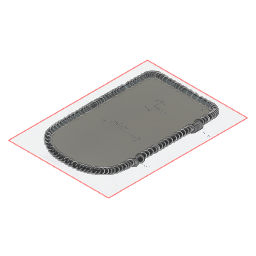
Uprint SE Screen (Autodesk Fusion 360 design; units mm, degrees)
Autodesk Fusion 360 part; units mm, degrees
sketch "Sketch1" plane through (0, 0, 0) normal (0, 0, 1) x (1, 0, 0)
  spline S0 degree 5 poles (-58.9, 25) (-58.8991, 25.1061) (-58.8974, 25.3171) (-58.8955, 25.6302) (-58.8941, 26.0406) (-58.8945, 26.5424) (-58.8966, 27.0343) (-58.9, 27.5189) (-58.9039, 28.0007) (-58.9072, 28.4862) (-58.9085, 28.9828) (-58.9065, 29.4974) (-58.9005, 30.0352) (-58.89, 30.598) (-58.8752, 31.1836) (-58.8572, 31.7866) (-58.8371, 32.4001) (-58.8162, 33.0168) (-58.7955, 33.6305) (-58.7759, 34.2371) (-58.7577, 34.8358) (-58.7409, 35.4283) (-58.725, 36.0179) (-58.7098, 36.6088) (-58.6948, 37.2055) (-58.6796, 37.8119) (-58.664, 38.431) (-58.648, 39.0645) (-58.6317, 39.7131) (-58.6152, 40.3763) (-58.5986, 41.052) (-58.5823, 41.7369) (-58.5663, 42.4263) (-58.5507, 43.1148) (-58.5357, 43.7974) (-58.5213, 44.4704) (-58.5075, 45.1325) (-58.4941, 45.7852) (-58.4811, 46.4341) (-58.468, 47.0889) (-58.4547, 47.7617) (-58.4408, 48.465) (-58.4259, 49.2109) (-58.41, 50.0087) (-58.3927, 50.8643) (-58.374, 51.7776) (-58.3541, 52.7428) (-58.3331, 53.7495) (-58.3114, 54.784) (-58.2892, 55.8308) (-58.2669, 56.8734) (-58.245, 57.8958) (-58.2238, 58.8838) (-58.2036, 59.8262) (-58.1848, 60.7157) (-58.1675, 61.5508) (-58.152, 62.335) (-58.1381, 63.0753) (-58.1258, 63.7812) (-58.1149, 64.4636) (-58.105, 65.134) (-58.0958, 65.8026) (-58.0865, 66.4778) (-58.0763, 67.1655) (-58.0646, 67.8691) (-58.0505, 68.59) (-58.0335, 69.3277) (-58.0133, 70.0802) (-57.9898, 70.8439) (-57.9634, 71.614) (-57.935, 72.385) (-57.9056, 73.1508) (-57.8763, 73.9064) (-57.848, 74.6475) (-57.8215, 75.3718) (-57.797, 76.0795) (-57.7742, 76.7738) (-57.7519, 77.4617) (-57.7287, 78.1521) (-57.7029, 78.8535) (-57.6729, 79.5733) (-57.6376, 80.3151) (-57.5967, 81.0775) (-57.5509, 81.8521) (-57.5019, 82.6224) (-57.4523, 83.3673) (-57.4046, 84.0651) (-57.3604, 84.697) (-57.3203, 85.2508) (-57.283, 85.7243) (-57.2445, 86.1299) (-57.1983, 86.4936) (-57.1374, 86.8447) (-57.0551, 87.2099) (-56.9468, 87.6027) (-56.8104, 88.0233) (-56.6459, 88.4642) (-56.4556, 88.9133) (-56.2433, 89.3591) (-56.0145, 89.7937) (-55.7743, 90.2123) (-55.5264, 90.6131) (-55.2717, 90.9968) (-55.0062, 91.367) (-54.7219, 91.729) (-54.4103, 92.0876) (-54.0646, 92.4458) (-53.6834, 92.803) (-53.273, 93.1523) (-52.8457, 93.4836) (-52.4159, 93.7859) (-51.9969, 94.0505) (-51.5979, 94.2734) (-51.2203, 94.4589) (-50.8589, 94.617) (-50.5057, 94.7597) (-50.1522, 94.897) (-49.7935, 95.0325) (-49.4276, 95.1645) (-49.0539, 95.2878) (-48.6727, 95.3967) (-48.283, 95.4865) (-47.8829, 95.5546) (-47.4692, 95.6002) (-47.0375, 95.6245) (-46.5821, 95.6312) (-46.0967, 95.6255) (-45.5763, 95.6131) (-45.018, 95.5995) (-44.4229, 95.5887) (-43.7967, 95.5829) (-43.1487, 95.5823) (-42.4895, 95.5859) (-41.8296, 95.592) (-41.1776, 95.5987) (-40.5384, 95.6041) (-39.9114, 95.6075) (-39.2909, 95.6084) (-38.6684, 95.6073) (-38.0341, 95.6047) (-37.3782, 95.6016) (-36.6931, 95.5986) (-35.975, 95.5963) (-35.2244, 95.5951) (-34.4448, 95.5949) (-33.6424, 95.5955) (-32.8245, 95.5967) (-31.9988, 95.5983) (-31.1729, 95.5998) (-30.3528, 95.601) (-29.5422, 95.6018) (-28.7429, 95.6021) (-27.955, 95.602) (-27.1781, 95.6016) (-26.4112, 95.601) (-25.6539, 95.6004) (-24.9064, 95.5999) (-24.1708, 95.5996) (-23.4507, 95.5995) (-22.7508, 95.5995) (-22.0753, 95.5997) (-21.4272, 95.5998) (-20.8072, 95.6) (-20.2126, 95.6) (-19.6359, 95.6) (-19.0653, 95.5999) (-18.4875, 95.5998) (-17.8893, 95.5998) (-17.2605, 95.5999) (-16.5953, 95.6001) (-15.8952, 95.6004) (-15.1686, 95.6008) (-14.4278, 95.601) (-13.6868, 95.601) (-12.9593, 95.6008) (-12.2558, 95.6003) (-11.582, 95.5996) (-10.9355, 95.5987) (-10.3068, 95.5979) (-9.6818, 95.5975) (-9.0444, 95.5977) (-8.3784, 95.5985) (-7.6701, 95.6002) (-6.911, 95.6026) (-6.0991, 95.6053) (-5.2378, 95.608) (-4.3344, 95.6102) (-3.3988, 95.6114) (-2.4427, 95.611) (-1.4776, 95.6086) (-0.5141, 95.6041) (0.4394, 95.5971) (1.3784, 95.5879) (2.3025, 95.5767) (3.2141, 95.5642) (4.1179, 95.5509) (5.0199, 95.5375) (5.9262, 95.5248) (6.8428, 95.5134) (7.7742, 95.5038) (8.7225, 95.4964) (9.687, 95.4914) (10.6632, 95.4887) (11.6446, 95.4879) (12.6231, 95.4888) (13.59, 95.4909) (14.537, 95.4935) (15.4567, 95.4963) (16.3436, 95.4987) (17.1952, 95.5005) (18.0128, 95.5015) (18.8017, 95.5018) (19.5702, 95.5014) (20.3282, 95.5008) (21.0862, 95.5001) (21.854, 95.4996) (22.6393, 95.4997) (23.4469, 95.5003) (24.2771, 95.5013) (25.1257, 95.5027) (25.9855, 95.5039) (26.8472, 95.5047) (27.7003, 95.5047) (28.5345, 95.5038) (29.3406, 95.5018) (30.1117, 95.4989) (30.8441, 95.4957) (31.538, 95.4929) (32.1959, 95.4912) (32.8216, 95.4916) (33.4196, 95.4943) (33.9936, 95.4995) (34.5453, 95.5063) (35.0741, 95.5132) (35.5782, 95.5177) (36.0567, 95.5163) (36.5115, 95.5039) (36.9493, 95.4745) (37.3833, 95.4202) (37.8291, 95.333) (38.3017, 95.2056) (38.8111, 95.0327) (39.3585, 94.8124) (39.935, 94.5462) (40.5255, 94.2385) (41.1116, 93.8957) (41.6747, 93.5252) (42.1988, 93.1351) (42.6737, 92.7332) (43.0977, 92.3261) (43.4746, 91.9191) (43.812, 91.5158) (44.1187, 91.1171) (44.4032, 90.7213) (44.6708, 90.3232) (44.9238, 89.9156) (45.1622, 89.4916) (45.385, 89.0467) (45.5901, 88.5811) (45.776, 88.102) (45.9413, 87.6203) (46.085, 87.1473) (46.2066, 86.6909) (46.3064, 86.2521) (46.3854, 85.8217) (46.4451, 85.385) (46.488, 84.9274) (46.5174, 84.4389) (46.5373, 83.9205) (46.5522, 83.3834) (46.5666, 82.8427) (46.5844, 82.3125) (46.6083, 81.8007) (46.6394, 81.303) (46.6765, 80.8014) (46.7175, 80.2727) (46.7595, 79.6944) (46.7993, 79.0515) (46.8342, 78.3428) (46.8624, 77.5884) (46.883, 76.8218) (46.896, 76.0823) (46.902, 75.407) (46.9025, 74.8232) (46.8993, 74.3408) (46.8949, 73.9426) (46.8923, 73.5835) (46.894, 73.209) (46.9016, 72.7699) (46.9155, 72.2407) (46.9341, 71.628) (46.955, 70.9576) (46.9753, 70.266) (46.9921, 69.5896) (47.0034, 68.956) (47.0086, 68.3729) (47.0085, 67.8217) (47.0053, 67.2706) (47.0015, 66.6843) (46.9991, 66.0356) (46.9997, 65.3148) (47.0031, 64.5426) (47.0074, 63.7742) (47.0102, 63.0768) (47.0093, 62.5129) (47.0042, 62.1193) (46.9969, 61.8927) (46.9928, 61.7611) (47.0033, 61.6066) (47.0613, 61.4198) (47.1962, 61.277) (47.3618, 61.2248) (47.5085, 61.2586) (47.6834, 61.3051) (47.9192, 61.3124) (48.1786, 61.2985) (48.4167, 61.2947) (48.6267, 61.3024) (48.8271, 61.3015) (49.0325, 61.2679) (49.2464, 61.1849) (49.4586, 61.0601) (49.6507, 60.9219) (49.8171, 60.7893) (49.9778, 60.6523) (50.1486, 60.4921) (50.3103, 60.302) (50.4273, 60.0853) (50.4851, 59.8481) (50.499, 59.5958) (50.4927, 59.3302) (50.4827, 59.0468) (50.4778, 58.7398) (50.4808, 58.4083) (50.4892, 58.062) (50.4986, 57.7133) (50.5044, 57.3717) (50.5051, 57.0346) (50.5025, 56.6907) (50.4991, 56.3279) (50.4971, 55.9403) (50.4971, 55.5336) (50.4985, 55.1182) (50.5005, 54.7044) (50.502, 54.2961) (50.5025, 53.8875) (50.5016, 53.4717) (50.4998, 53.0458) (50.4978, 52.619) (50.497, 52.217) (50.4982, 51.8654) (50.5012, 51.5782) (50.5035, 51.3379) (50.5, 51.1015) (50.4832, 50.8434) (50.4434, 50.5959) (50.3719, 50.4086) (50.2676, 50.2745) (50.136, 50.1274) (49.9766, 49.9477) (49.7839, 49.7722) (49.5625, 49.6389) (49.3337, 49.5548) (49.1161, 49.5105) (48.9022, 49.4942) (48.6701, 49.4956) (48.428, 49.4998) (48.2166, 49.4921) (48.049, 49.4786) (47.8707, 49.4997) (47.6602, 49.5468) (47.4901, 49.5171) (47.4063, 49.3709) (47.3746, 49.1931) (47.365, 48.9995) (47.3644, 48.7374) (47.3658, 48.3831) (47.3664, 47.9629) (47.3657, 47.52) (47.3647, 47.0967) (47.3641, 46.7046) (47.3641, 46.3254) (47.3647, 45.9286) (47.366, 45.4818) (47.3681, 44.9668) (47.3715, 44.3815) (47.3767, 43.7341) (47.3842, 43.04) (47.3942, 42.3175) (47.4069, 41.5843) (47.4218, 40.8525) (47.4381, 40.1286) (47.4548, 39.4143) (47.4709, 38.7082) (47.4852, 38.0068) (47.4968, 37.3058) (47.5051, 36.6015) (47.51, 35.8917) (47.5117, 35.1767) (47.5108, 34.458) (47.5082, 33.738) (47.5047, 33.0197) (47.5011, 32.3059) (47.4983, 31.5991) (47.4964, 30.9006) (47.4957, 30.2102) (47.496, 29.5273) (47.497, 28.8499) (47.4985, 28.1758) (47.4999, 27.5022) (47.501, 26.8262) (47.5017, 26.1447) (47.502, 25.4547) (47.5018, 24.7536) (47.5013, 24.0392) (47.5007, 23.3099) (47.5, 22.565) (47.4995, 21.8047) (47.4991, 21.0302) (47.499, 20.244) (47.499, 19.449) (47.4992, 18.6484) (47.4995, 17.8458) (47.4998, 17.0446) (47.5001, 16.2478) (47.5003, 15.4577) (47.5004, 14.676) (47.5004, 13.9033) (47.5004, 13.1402) (47.5003, 12.3864) (47.5001, 11.6415) (47.5, 10.905) (47.4999, 10.1763) (47.4999, 9.455) (47.4998, 8.7407) (47.4999, 8.033) (47.4999, 7.3317) (47.4999, 6.6362) (47.5, 5.9459) (47.5, 5.2598) (47.5001, 4.5769) (47.5001, 3.8955) (47.5001, 3.2141) (47.5, 2.5309) (47.5, 1.8444) (47.5, 1.1529) (47.5, 0.4552) (47.5, -0.2496) (47.4999, -0.9622) (47.4999, -1.6832) (47.4999, -2.4127) (47.5, -3.0032) (47.5, -3.4501) (47.5, -3.7497) (47.5, -3.9) knots 0 0 0 0 0 0 0.00222222 0.00444444 0.00666667 0.00888889 0.01111111 0.01333333 0.01555556 0.01777778 0.02 0.02222222 0.02444444 0.02666667 0.02888889 0.03111111 0.03333333 0.03555556 0.03777778 0.04 0.04222222 0.04444444 0.04666667 0.04888889 0.05111111 0.05333333 0.05555556 0.05777778 0.06 0.06222222 0.06444444 0.06666667 0.06888889 0.07111111 0.07333333 0.07555556 0.07777778 0.08 0.08222222 0.08444444 0.08666667 0.08888889 0.09111111 0.09333333 0.09555556 0.09777778 0.1 0.10222222 0.10444444 0.10666667 0.10888889 0.11111111 0.11333333 0.11555556 0.11777778 0.12 0.12222222 0.12444444 0.12666667 0.12888889 0.13111111 0.13333333 0.13555556 0.13777778 0.14 0.14222222 0.14444444 0.14666667 0.14888889 0.15111111 0.15333333 0.15555556 0.15777778 0.16 0.16222222 0.16444444 0.16666667 0.16888889 0.17111111 0.17333333 0.17555556 0.17777778 0.18 0.18222222 0.18444444 0.18666667 0.18888889 0.19111111 0.19333333 0.19555556 0.19777778 0.2 0.20222222 0.20444444 0.20666667 0.20888889 0.21111111 0.21333333 0.21555556 0.21777778 0.22 0.22222222 0.22444444 0.22666667 0.22888889 0.23111111 0.23333333 0.23555556 0.23777778 0.24 0.24222222 0.24444444 0.24666667 0.24888889 0.25111111 0.25333333 0.25555556 0.25777778 0.26 0.26222222 0.26444444 0.26666667 0.26888889 0.27111111 0.27333333 0.27555556 0.27777778 0.28 0.28222222 0.28444444 0.28666667 0.28888889 0.29111111 0.29333333 0.29555556 0.29777778 0.3 0.30222222 0.30444444 0.30666667 0.30888889 0.31111111 0.31333333 0.31555556 0.31777778 0.32 0.32222222 0.32444444 0.32666667 0.32888889 0.33111111 0.33333333 0.33555556 0.33777778 0.34 0.34222222 0.34444444 0.34666667 0.34888889 0.35111111 0.35333333 0.35555556 0.35777778 0.36 0.36222222 0.36444444 0.36666667 0.36888889 0.37111111 0.37333333 0.37555556 0.37777778 0.38 0.38222222 0.38444444 0.38666667 0.38888889 0.39111111 0.39333333 0.39555556 0.39777778 0.4 0.40222222 0.40444444 0.40666667 0.40888889 0.41111111 0.41333333 0.41555556 0.41777778 0.42 0.42222222 0.42444444 0.42666667 0.42888889 0.43111111 0.43333333 0.43555556 0.43777778 0.44 0.44222222 0.44444444 0.44666667 0.44888889 0.45111111 0.45333333 0.45555556 0.45777778 0.46 0.46222222 0.46444444 0.46666667 0.46888889 0.47111111 0.47333333 0.47555556 0.47777778 0.48 0.48222222 0.48444444 0.48666667 0.48888889 0.49111111 0.49333333 0.49555556 0.49777778 0.5 0.50222222 0.50444444 0.50666667 0.50888889 0.51111111 0.51333333 0.51555556 0.51777778 0.52 0.52222222 0.52444444 0.52666667 0.52888889 0.53111111 0.53333333 0.53555556 0.53777778 0.54 0.54222222 0.54444444 0.54666667 0.54888889 0.55111111 0.55333333 0.55555556 0.55777778 0.56 0.56222222 0.56444444 0.56666667 0.56888889 0.57111111 0.57333333 0.57555556 0.57777778 0.58 0.58222222 0.58444444 0.58666667 0.58888889 0.59111111 0.59333333 0.59555556 0.59777778 0.6 0.60222222 0.60444444 0.60666667 0.60888889 0.61111111 0.61333333 0.61555556 0.61777778 0.62 0.62222222 0.62444444 0.62666667 0.62888889 0.63111111 0.63333333 0.63555556 0.63777778 0.64 0.64222222 0.64444444 0.64666667 0.64888889 0.65111111 0.65333333 0.65555556 0.65777778 0.66 0.66222222 0.66444444 0.66666667 0.66888889 0.67111111 0.67333333 0.67555556 0.67777778 0.68 0.68222222 0.68444444 0.68666667 0.68888889 0.69111111 0.69333333 0.69555556 0.69777778 0.7 0.70222222 0.70444444 0.70666667 0.70888889 0.71111111 0.71333333 0.71555556 0.71777778 0.72 0.72222222 0.72444444 0.72666667 0.72888889 0.73111111 0.73333333 0.73555556 0.73777778 0.74 0.74222222 0.74444444 0.74666667 0.74888889 0.75111111 0.75333333 0.75555556 0.75777778 0.76 0.76222222 0.76444444 0.76666667 0.76888889 0.77111111 0.77333333 0.77555556 0.77777778 0.78 0.78222222 0.78444444 0.78666667 0.78888889 0.79111111 0.79333333 0.79555556 0.79777778 0.8 0.80222222 0.80444444 0.80666667 0.80888889 0.81111111 0.81333333 0.81555556 0.81777778 0.82 0.82222222 0.82444444 0.82666667 0.82888889 0.83111111 0.83333333 0.83555556 0.83777778 0.84 0.84222222 0.84444444 0.84666667 0.84888889 0.85111111 0.85333333 0.85555556 0.85777778 0.86 0.86222222 0.86444444 0.86666667 0.86888889 0.87111111 0.87333333 0.87555556 0.87777778 0.88 0.88222222 0.88444444 0.88666667 0.88888889 0.89111111 0.89333333 0.89555556 0.89777778 0.9 0.90222222 0.90444444 0.90666667 0.90888889 0.91111111 0.91333333 0.91555556 0.91777778 0.92 0.92222222 0.92444444 0.92666667 0.92888889 0.93111111 0.93333333 0.93555556 0.93777778 0.94 0.94222222 0.94444444 0.94666667 0.94888889 0.95111111 0.95333333 0.95555556 0.95777778 0.96 0.96222222 0.96444444 0.96666667 0.96888889 0.97111111 0.97333333 0.97555556 0.97777778 0.98 0.98222222 0.98444444 0.98666667 0.98888889 0.99111111 0.99333333 0.99555556 0.99777778 1 1 1 1 1 1
  spline S1 degree 5 poles (47.5, -3.9) (47.5002, -4.0074) (47.5004, -4.2192) (47.5007, -4.5278) (47.5008, -4.9212) (47.5005, -5.3852) (47.5, -5.8286) (47.4993, -6.266) (47.4989, -6.7214) (47.499, -7.2219) (47.4998, -7.7922) (47.5014, -8.4486) (47.5033, -9.1934) (47.505, -10.0178) (47.5059, -10.9052) (47.5054, -11.8343) (47.5031, -12.7821) (47.4993, -13.7267) (47.4943, -14.651) (47.4893, -15.5448) (47.4857, -16.4032) (47.4848, -17.2266) (47.4875, -18.019) (47.4942, -18.7876) (47.5043, -19.5418) (47.5158, -20.2924) (47.5258, -21.0505) (47.5311, -21.8252) (47.5289, -22.6223) (47.518, -23.4424) (47.4991, -24.2788) (47.4761, -25.116) (47.4563, -25.9285) (47.4476, -26.6867) (47.4556, -27.3626) (47.4802, -27.9362) (47.5143, -28.4005) (47.5372, -28.7694) (47.5247, -29.0747) (47.4753, -29.3467) (47.4461, -29.5956) (47.5241, -29.8048) (47.6869, -29.9258) (47.8228, -29.9125) (47.9727, -29.8835) (48.172, -29.9002) (48.387, -29.9099) (48.5473, -29.8972) (48.6603, -29.8852) (48.8636, -29.9267) (49.1105, -29.9993) (49.3114, -30.0724) (49.4998, -30.1893) (49.725, -30.376) (49.9562, -30.5656) (50.1385, -30.7045) (50.2559, -30.8868) (50.3288, -31.2974) (50.3802, -32.0586) (50.4225, -33.1649) (50.4612, -34.5297) (50.496, -36.011) (50.5234, -37.4445) (50.538, -38.6742) (50.5345, -39.5834) (50.5097, -40.1278) (50.4642, -40.3612) (50.4051, -40.4816) (50.3307, -40.6727) (50.211, -40.9136) (50.0306, -41.1197) (49.8276, -41.2804) (49.6424, -41.4205) (49.4578, -41.5637) (49.2335, -41.7171) (48.9692, -41.8565) (48.6907, -41.9432) (48.4081, -41.9544) (48.1102, -41.9021) (47.8027, -41.8447) (47.5358, -41.8967) (47.3654, -42.1518) (47.2964, -42.5726) (47.2926, -43.0345) (47.307, -43.4179) (47.3115, -43.71) (47.3036, -44.003) (47.2899, -44.4042) (47.2748, -44.9588) (47.2589, -45.6525) (47.2407, -46.4367) (47.2181, -47.2464) (47.1891, -48.0205) (47.1536, -48.7238) (47.1132, -49.3556) (47.0706, -49.9359) (47.0281, -50.4964) (46.9874, -51.0702) (46.9478, -51.6811) (46.9061, -52.3366) (46.858, -53.0338) (46.799, -53.7627) (46.7252, -54.51) (46.635, -55.2628) (46.5295, -56.013) (46.4126, -56.7571) (46.2889, -57.4951) (46.1633, -58.2293) (46.039, -58.9632) (45.9167, -59.7003) (45.7932, -60.4432) (45.6617, -61.1931) (45.514, -61.9499) (45.3416, -62.7122) (45.1375, -63.4774) (44.8973, -64.2417) (44.6215, -64.9999) (44.3152, -65.746) (43.9865, -66.4738) (43.6443, -67.1774) (43.2973, -67.8519) (42.9519, -68.4943) (42.6107, -69.1039) (42.2709, -69.683) (41.9266, -70.2358) (41.5703, -70.768) (41.1949, -71.2857) (40.7949, -71.7946) (40.3694, -72.2994) (39.9203, -72.8036) (39.4516, -73.3097) (38.968, -73.8191) (38.4734, -74.3323) (37.9699, -74.849) (37.4564, -75.3683) (36.9306, -75.8885) (36.3897, -76.4076) (35.8314, -76.9228) (35.2553, -77.4314) (34.6635, -77.93) (34.0618, -78.4153) (33.4574, -78.8843) (32.8577, -79.3348) (32.2686, -79.7658) (31.6931, -80.1779) (31.1295, -80.5738) (30.5705, -80.9587) (30.0057, -81.3387) (29.4238, -81.7199) (28.8151, -82.1071) (28.1733, -82.5031) (27.4985, -82.9067) (26.7971, -83.3135) (26.0793, -83.7165) (25.3575, -84.1082) (24.6441, -84.481) (23.9492, -84.8289) (23.2791, -85.1487) (22.6341, -85.4408) (22.0103, -85.7085) (21.4007, -85.9566) (20.7968, -86.1908) (20.19, -86.4164) (19.573, -86.637) (18.9408, -86.8548) (18.2899, -87.0705) (17.6186, -87.2839) (16.9269, -87.4944) (16.2161, -87.701) (15.4888, -87.9034) (14.7483, -88.101) (13.9979, -88.2936) (13.2408, -88.4805) (12.4785, -88.6612) (11.7112, -88.8343) (10.9365, -88.9983) (10.1502, -89.1512) (9.3474, -89.2908) (8.5234, -89.4153) (7.6751, -89.5233) (6.8014, -89.6141) (5.9045, -89.6878) (4.9909, -89.7461) (4.0696, -89.7912) (3.1509, -89.826) (2.2448, -89.8535) (1.3599, -89.8765) (0.5018, -89.8975) (-0.3284, -89.9179) (-1.1351, -89.9381) (-1.9273, -89.9576) (-2.7164, -89.9751) (-3.5138, -89.9893) (-4.3297, -89.9986) (-5.1708, -90.002) (-6.0382, -89.999) (-6.9265, -89.99) (-7.8265, -89.9761) (-8.7265, -89.9584) (-9.6143, -89.9382) (-10.4794, -89.9167) (-11.3144, -89.8945) (-12.1173, -89.8716) (-12.8928, -89.8471) (-13.6493, -89.8194) (-14.3975, -89.787) (-15.1481, -89.7481) (-15.9102, -89.7013) (-16.6885, -89.6456) (-17.4822, -89.5809) (-18.2862, -89.5076) (-19.0929, -89.4264) (-19.8938, -89.3382) (-20.6815, -89.2432) (-21.4509, -89.1417) (-22.2014, -89.0328) (-22.9369, -88.9152) (-23.6639, -88.7869) (-24.3906, -88.6455) (-25.1252, -88.4889) (-25.875, -88.3147) (-26.6445, -88.121) (-27.4355, -87.9065) (-28.2473, -87.67) (-29.0775, -87.4109) (-29.9227, -87.129) (-30.7786, -86.8244) (-31.6411, -86.4976) (-32.5065, -86.1496) (-33.3717, -85.7815) (-34.2342, -85.3947) (-35.0921, -84.9908) (-35.9439, -84.5712) (-36.7887, -84.1373) (-37.6256, -83.6903) (-38.4544, -83.2308) (-39.2748, -82.7594) (-40.0868, -82.2761) (-40.8904, -81.7808) (-41.6858, -81.2732) (-42.4727, -80.7532) (-43.2507, -80.2208) (-44.0192, -79.6762) (-44.777, -79.1201) (-45.5226, -78.5534) (-46.254, -77.9774) (-46.9693, -77.3936) (-47.6666, -76.8031) (-48.3442, -76.207) (-49.0006, -75.6059) (-49.6349, -74.9998) (-50.2469, -74.3882) (-50.8366, -73.77) (-51.4044, -73.1439) (-51.9505, -72.5086) (-52.475, -71.8631) (-52.9773, -71.2067) (-53.4562, -70.5398) (-53.9097, -69.8634) (-54.335, -69.1793) (-54.7299, -68.4892) (-55.0924, -67.795) (-55.4214, -67.0977) (-55.7175, -66.3976) (-55.9831, -65.694) (-56.2222, -64.9846) (-56.4397, -64.2672) (-56.6408, -63.5391) (-56.83, -62.7982) (-57.0109, -62.0432) (-57.1851, -61.2745) (-57.3524, -60.4933) (-57.5115, -59.7022) (-57.6602, -58.9041) (-57.7964, -58.1018) (-57.9184, -57.298) (-58.0252, -56.4947) (-58.1176, -55.6927) (-58.197, -54.8921) (-58.2657, -54.0927) (-58.3262, -53.2939) (-58.3812, -52.4955) (-58.4329, -51.6976) (-58.4827, -50.9011) (-58.5313, -50.1076) (-58.5788, -49.3188) (-58.6251, -48.5364) (-58.6695, -47.7615) (-58.7116, -46.9945) (-58.751, -46.2344) (-58.7873, -45.4785) (-58.8206, -44.7237) (-58.8509, -43.9658) (-58.8783, -43.2011) (-58.903, -42.426) (-58.9251, -41.6379) (-58.9446, -40.8354) (-58.9615, -40.0183) (-58.9758, -39.1872) (-58.9875, -38.3437) (-58.9966, -37.4898) (-59.0031, -36.628) (-59.0073, -35.7611) (-59.0092, -34.892) (-59.0093, -34.0235) (-59.008, -33.1582) (-59.0054, -32.2983) (-59.0021, -31.4453) (-58.9982, -30.6001) (-58.9941, -29.7625) (-58.9897, -28.9315) (-58.9854, -28.1051) (-58.9812, -27.2808) (-58.9771, -26.4554) (-58.9736, -25.6254) (-58.9707, -24.7871) (-58.969, -23.9365) (-58.9689, -23.0701) (-58.971, -22.1851) (-58.9757, -21.2805) (-58.9833, -20.357) (-58.9938, -19.4181) (-59.0071, -18.4703) (-59.0226, -17.5241) (-59.0394, -16.5928) (-59.0564, -15.6908) (-59.0724, -14.8311) (-59.0864, -14.0236) (-59.0974, -13.273) (-59.105, -12.5769) (-59.1088, -11.9232) (-59.1094, -11.2919) (-59.1073, -10.6604) (-59.1034, -10.0076) (-59.0987, -9.3182) (-59.0943, -8.5877) (-59.0912, -7.8252) (-59.0902, -7.0473) (-59.0916, -6.2749) (-59.0955, -5.5285) (-59.1013, -4.8238) (-59.1076, -4.1673) (-59.1124, -3.5534) (-59.1134, -2.9695) (-59.1088, -2.3994) (-59.0975, -1.8271) (-59.0797, -1.2415) (-59.0573, -0.6388) (-59.0332, -0.0206) (-59.0106, 0.6065) (-58.9925, 1.2324) (-58.9811, 1.8442) (-58.9776, 2.4276) (-58.9824, 2.9683) (-58.9955, 3.4536) (-59.0167, 3.8737) (-59.04, 4.1535) (-59.061, 4.3311) (-59.0766, 4.4351) (-59.0848, 4.4835) knots 0 0 0 0 0 0 0.0028169 0.0056338 0.0084507 0.01126761 0.01408451 0.01690141 0.01971831 0.02253521 0.02535211 0.02816901 0.03098592 0.03380282 0.03661972 0.03943662 0.04225352 0.04507042 0.04788732 0.05070423 0.05352113 0.05633803 0.05915493 0.06197183 0.06478873 0.06760563 0.07042254 0.07323944 0.07605634 0.07887324 0.08169014 0.08450704 0.08732394 0.09014085 0.09295775 0.09577465 0.09859155 0.10140845 0.10422535 0.10704225 0.10985915 0.11267606 0.11549296 0.11830986 0.12112676 0.12394366 0.12676056 0.12957746 0.13239437 0.13521127 0.13802817 0.14084507 0.14366197 0.14647887 0.14929577 0.15211268 0.15492958 0.15774648 0.16056338 0.16338028 0.16619718 0.16901408 0.17183099 0.17464789 0.17746479 0.18028169 0.18309859 0.18591549 0.18873239 0.1915493 0.1943662 0.1971831 0.2 0.2028169 0.2056338 0.2084507 0.21126761 0.21408451 0.21690141 0.21971831 0.22253521 0.22535211 0.22816901 0.23098592 0.23380282 0.23661972 0.23943662 0.24225352 0.24507042 0.24788732 0.25070423 0.25352113 0.25633803 0.25915493 0.26197183 0.26478873 0.26760563 0.27042254 0.27323944 0.27605634 0.27887324 0.28169014 0.28450704 0.28732394 0.29014085 0.29295775 0.29577465 0.29859155 0.30140845 0.30422535 0.30704225 0.30985915 0.31267606 0.31549296 0.31830986 0.32112676 0.32394366 0.32676056 0.32957746 0.33239437 0.33521127 0.33802817 0.34084507 0.34366197 0.34647887 0.34929577 0.35211268 0.35492958 0.35774648 0.36056338 0.36338028 0.36619718 0.36901408 0.37183099 0.37464789 0.37746479 0.38028169 0.38309859 0.38591549 0.38873239 0.3915493 0.3943662 0.3971831 0.4 0.4028169 0.4056338 0.4084507 0.41126761 0.41408451 0.41690141 0.41971831 0.42253521 0.42535211 0.42816901 0.43098592 0.43380282 0.43661972 0.43943662 0.44225352 0.44507042 0.44788732 0.45070423 0.45352113 0.45633803 0.45915493 0.46197183 0.46478873 0.46760563 0.47042254 0.47323944 0.47605634 0.47887324 0.48169014 0.48450704 0.48732394 0.49014085 0.49295775 0.49577465 0.49859155 0.50140845 0.50422535 0.50704225 0.50985915 0.51267606 0.51549296 0.51830986 0.52112676 0.52394366 0.52676056 0.52957746 0.53239437 0.53521127 0.53802817 0.54084507 0.54366197 0.54647887 0.54929577 0.55211268 0.55492958 0.55774648 0.56056338 0.56338028 0.56619718 0.56901408 0.57183099 0.57464789 0.57746479 0.58028169 0.58309859 0.58591549 0.58873239 0.5915493 0.5943662 0.5971831 0.6 0.6028169 0.6056338 0.6084507 0.61126761 0.61408451 0.61690141 0.61971831 0.62253521 0.62535211 0.62816901 0.63098592 0.63380282 0.63661972 0.63943662 0.64225352 0.64507042 0.64788732 0.65070423 0.65352113 0.65633803 0.65915493 0.66197183 0.66478873 0.66760563 0.67042254 0.67323944 0.67605634 0.67887324 0.68169014 0.68450704 0.68732394 0.69014085 0.69295775 0.69577465 0.69859155 0.70140845 0.70422535 0.70704225 0.70985915 0.71267606 0.71549296 0.71830986 0.72112676 0.72394366 0.72676056 0.72957746 0.73239437 0.73521127 0.73802817 0.74084507 0.74366197 0.74647887 0.74929577 0.75211268 0.75492958 0.75774648 0.76056338 0.76338028 0.76619718 0.76901408 0.77183099 0.77464789 0.77746479 0.78028169 0.78309859 0.78591549 0.78873239 0.7915493 0.7943662 0.7971831 0.8 0.8028169 0.8056338 0.8084507 0.81126761 0.81408451 0.81690141 0.81971831 0.82253521 0.82535211 0.82816901 0.83098592 0.83380282 0.83661972 0.83943662 0.84225352 0.84507042 0.84788732 0.85070423 0.85352113 0.85633803 0.85915493 0.86197183 0.86478873 0.86760563 0.87042254 0.87323944 0.87605634 0.87887324 0.88169014 0.88450704 0.88732394 0.89014085 0.89295775 0.89577465 0.89859155 0.90140845 0.90422535 0.90704225 0.90985915 0.91267606 0.91549296 0.91830986 0.92112676 0.92394366 0.92676056 0.92957746 0.93239437 0.93521127 0.93802817 0.94084507 0.94366197 0.94647887 0.94929577 0.95211268 0.95492958 0.95774648 0.96056338 0.96338028 0.96619718 0.96901408 0.97183099 0.97464789 0.97746479 0.98028169 0.98309859 0.98591549 0.98873239 0.9915493 0.9943662 0.9971831 1 1 1 1 1 1
  line L0 (47, 61.7) -> (47.3653, 48.8491)
  line L1 (47.3019, -42.7439) -> (47.5, -29.7)
  spline S2 degree 5 poles (-58.9, 25) (-58.895, 24.8412) (-58.8857, 24.5256) (-58.8736, 24.0587) (-58.8612, 23.4489) (-58.8517, 22.7075) (-58.8482, 21.9855) (-58.85, 21.2792) (-58.8564, 20.5829) (-58.866, 19.8873) (-58.877, 19.1809) (-58.8877, 18.4527) (-58.8963, 17.6949) (-58.9019, 16.905) (-58.9042, 16.0887) (-58.9038, 15.2615) (-58.902, 14.4428) (-58.9001, 13.6529) (-58.8994, 12.9077) (-58.9003, 12.2154) (-58.9025, 11.5707) (-58.9044, 10.9564) (-58.9045, 10.3505) (-58.9016, 9.7325) (-58.8958, 9.0894) (-58.8889, 8.4226) (-58.8839, 7.7452) (-58.8847, 7.0768) (-58.8953, 6.4391) (-58.9187, 5.8507) (-58.957, 5.323) (-59.0002, 4.9536) (-59.0397, 4.7068) (-59.0692, 4.5557) (-59.0848, 4.4835) knots 0 0 0 0 0 0 0.033333 0.066667 0.1 0.133333 0.166667 0.2 0.233333 0.266667 0.3 0.333333 0.366667 0.4 0.433333 0.466667 0.5 0.533333 0.566667 0.6 0.633333 0.666667 0.7 0.733333 0.766667 0.8 0.833333 0.866667 0.9 0.933333 0.966667 1 1 1 1 1 1
  point P0 (-58.9, 27.5)
  point P1 (-58.9, 30)
  point P2 (-58.8, 33.5)
  point P3 (-58.7, 37)
  point P4 (-58.6, 41)
  point P5 (-58.5, 45.5)
  point P6 (-58.4, 50.5)
  point P7 (-58.2, 60)
  point P8 (-58.1, 65.5)
  point P9 (-58, 70.5)
  point P10 (-57.8, 76)
  point P11 (-57.6, 81)
  point P12 (-57.3, 85.5)
  point P13 (-57.1, 87)
  point P14 (-56.5, 88.8)
  point P15 (-55.4, 90.8)
  point P16 (-54, 92.5)
  point P17 (-51.9, 94.1)
  point P18 (-50.4, 94.8)
  point P19 (-49, 95.3)
  point P20 (-47.4, 95.6)
  point P21 (-45, 95.6)
  point P22 (-41, 95.6)
  point P23 (-37, 95.6)
  point P24 (-31, 95.6)
  point P25 (-25, 95.6)
  point P26 (-20.5, 95.6)
  point P27 (-17, 95.6)
  point P28 (-12, 95.6)
  point P29 (-7.8, 95.6)
  point P30 (0, 95.6)
  point P31 (8.3, 95.5)
  point P32 (17, 95.5)
  point P33 (23, 95.5)
  point P34 (29.8, 95.5)
  point P35 (34, 95.5)
  point P36 (36.5, 95.5)
  point P37 (38.6, 95.1)
  point P38 (42.1, 93.2)
  point P39 (44.2, 91)
  point P40 (45.4, 89)
  point P41 (46.2, 86.7)
  point P42 (46.5, 84.7)
  point P43 (46.6, 82)
  point P44 (46.8, 79)
  point P45 (46.9, 74.5)
  point P46 (46.9, 72.9)
  point P47 (47, 69.1)
  point P48 (47, 65.5)
  point P49 (47, 62)
  point P50 (47, 61.7)
  point P51 (47.1, 61.4)
  point P52 (47.352, 61.2463)
  point P53 (47.644, 61.288)
  point P54 (48.2, 61.3)
  point P55 (48.7, 61.3)
  point P56 (49.1458, 61.2185)
  point P57 (49.6296, 60.9342)
  point P58 (50.0053, 60.6235)
  point P59 (50.3714, 60.1731)
  point P60 (50.4942, 59.5734)
  point P61 (50.4798, 58.7497)
  point P62 (50.5, 57.6)
  point P63 (50.5, 56.4)
  point P64 (50.5, 54.8)
  point P65 (50.5, 53.1)
  point P66 (50.5, 51.7)
  point P67 (50.4949, 51.0609)
  point P68 (50.4, 50.5)
  point P69 (50.2, 50.2)
  point P70 (49.8, 49.8)
  point P71 (49.2579, 49.5441)
  point P72 (48.7553, 49.4961)
  point P73 (48.2439, 49.4917)
  point P74 (47.9, 49.5)
  point P75 (47.5489, 49.5092)
  point P76 (47.4, 49.3)
  point P77 (47.3653, 48.8491)
  point P78 (47.3653, 47.3674)
  point P79 (47.3653, 45.7632)
  point P80 (47.4, 42)
  point P81 (47.5, 37)
  point P82 (47.5, 32)
  point P83 (47.5, 27.4)
  point P84 (47.5, 22.5)
  point P85 (47.5, 16.4)
  point P86 (47.5, 10.7)
  point P87 (47.5, 5.8)
  point P88 (47.5, 1.2)
  point P89 (47.5, -5.8)
  point P90 (47.5, -7.8)
  point P91 (47.5, -13.5)
  point P92 (47.5, -19.2)
  point P93 (47.5, -24.2)
  point P94 (47.5, -28.2)
  point P95 (47.5, -29.2)
  point P96 (47.5, -29.7)
  point P97 (47.7, -29.9)
  point P98 (47.9, -29.9)
  point P99 (48.2, -29.9)
  point P100 (48.5, -29.9)
  point P101 (48.7, -29.9)
  point P102 (49.1, -30)
  point P103 (49.5, -30.2)
  point P104 (50, -30.6)
  point P105 (50.3, -31.2)
  point P106 (50.5, -40.1)
  point P107 (50.4, -40.5)
  point P108 (50.2, -40.9)
  point P109 (49.8, -41.3)
  point P110 (49.4, -41.6)
  point P111 (48.8, -41.9)
  point P112 (48.1, -41.9)
  point P113 (47.5, -42)
  point P114 (47.3, -43.2)
  point P115 (47.3, -44.1)
  point P116 (47.2, -47.7)
  point P117 (47, -50.9)
  point P118 (46.7, -54.7)
  point P119 (46, -59.2)
  point P120 (45, -63.9)
  point P121 (43, -68.4)
  point P122 (41.1, -71.4)
  point P123 (38.6, -74.2)
  point P124 (35.4, -77.3)
  point P125 (31.8, -80.1)
  point P126 (28.5, -82.3)
  point P127 (24, -84.8)
  point P128 (20.5, -86.3)
  point P129 (16.9, -87.5)
  point P130 (12.3, -88.7)
  point P131 (6.9, -89.6)
  point P132 (0.4, -89.9)
  point P133 (-4.9, -90)
  point P134 (-11.1, -89.9)
  point P135 (-15.9, -89.7)
  point P136 (-21, -89.2)
  point P137 (-25.5, -88.4)
  point P138 (-31.1, -86.7)
  point P139 (-37.6, -83.7)
  point P140 (-43.7, -79.9)
  point P141 (-49, -75.6)
  point P142 (-52.9, -71.3)
  point P143 (-55.5, -66.9)
  point P144 (-56.9, -62.5)
  point P145 (-57.9, -57.4)
  point P146 (-58.4, -52.2)
  point P147 (-58.7, -47.2)
  point P148 (-58.9, -42.5)
  point P149 (-59, -37)
  point P150 (-59, -31)
  point P151 (-58.973, -25.4226)
  point P152 (-59, -19)
  point P153 (-59.1, -13)
  point P154 (-59.1, -9.5)
  point P155 (-59.1, -5)
  point P156 (-59.1, -2)
  point P157 (-59, 1)
  point P158 (-59, 3.5)
  point P159 (-58.8532, 20.9966)
  point P160 (-58.9, 17.1)
  point P161 (-58.9, 12.6)
  point P162 (-58.9, 9.6)
  point P163 (-58.9, 6.4)
  constraint coincident P50 L0.start
  constraint coincident P77 L0.end
  constraint coincident S1 L1.start
  constraint coincident P96 L1.end
extrude "Extrude1" add sketch "Sketch1" along normal blind 3 contours S0 S1 L0 L1 S2
extrude "Extrude2" add sketch "Sketch1" along normal blind 3 contours S1 L1
extrude "Extrude3" add sketch "Sketch1" along normal blind 3 contours S0 L0
extrude "Extrude4" cut sketch "Sketch1" along normal blind 1 contours S0 L0
extrude "Extrude5" cut sketch "Sketch1" along normal blind 1 contours S1 L1
named bodies: "Screen Cover"
